Autodesk Fusion 360 part; units mm, degrees
(part 6 of 11)
  spline S6 degree 5 poles (6.7301, -111.4554) (6.7368, -111.4652) (6.7506, -111.4847) (6.7724, -111.5129) (6.8034, -111.549) (6.8449, -111.592) (6.8883, -111.6333) (6.9329, -111.6738) (6.9782, -111.7138) (7.0239, -111.7534) (7.0701, -111.7926) (7.117, -111.8312) (7.1647, -111.8691) (7.2134, -111.9062) (7.263, -111.9424) (7.3134, -111.9779) (7.3646, -112.0127) (7.4164, -112.0469) (7.4687, -112.0806) (7.5214, -112.1138) (7.5747, -112.1465) (7.6286, -112.1787) (7.6829, -112.2103) (7.7379, -112.2413) (7.7934, -112.2717) (7.8494, -112.3016) (7.9059, -112.331) (7.9629, -112.3598) (8.0204, -112.3881) (8.0782, -112.4159) (8.1365, -112.4432) (8.1952, -112.47) (8.2544, -112.4963) (8.314, -112.5221) (8.374, -112.5473) (8.4344, -112.5721) (8.4952, -112.5964) (8.5564, -112.6201) (8.6179, -112.6434) (8.6798, -112.6662) (8.7421, -112.6885) (8.8047, -112.7103) (8.8677, -112.7316) (8.9311, -112.7524) (8.9947, -112.7727) (9.0587, -112.7926) (9.1231, -112.812) (9.1877, -112.8308) (9.2527, -112.8492) (9.318, -112.8672) (9.3836, -112.8846) (9.4494, -112.9015) (9.5156, -112.918) (9.5821, -112.934) (9.6488, -112.9495) (9.7158, -112.9646) (9.7831, -112.9791) (9.8507, -112.9932) (9.9186, -113.0068) (9.9866, -113.02) (10.055, -113.0326) (10.1236, -113.0448) (10.1925, -113.0565) (10.2615, -113.0678) (10.3309, -113.0785) (10.4004, -113.0888) (10.4702, -113.0986) (10.5403, -113.108) (10.6105, -113.1168) (10.6809, -113.1252) (10.7516, -113.1331) (10.8083, -113.1391) (10.851, -113.1434) (10.8794, -113.1461) (10.8937, -113.1475) knots 0 0 0 0 0 0 0.01428571 0.02857143 0.04285714 0.05714286 0.07142857 0.08571429 0.1 0.11428571 0.12857143 0.14285714 0.15714286 0.17142857 0.18571429 0.2 0.21428571 0.22857143 0.24285714 0.25714286 0.27142857 0.28571429 0.3 0.31428571 0.32857143 0.34285714 0.35714286 0.37142857 0.38571429 0.4 0.41428571 0.42857143 0.44285714 0.45714286 0.47142857 0.48571429 0.5 0.51428571 0.52857143 0.54285714 0.55714286 0.57142857 0.58571429 0.6 0.61428571 0.62857143 0.64285714 0.65714286 0.67142857 0.68571429 0.7 0.71428571 0.72857143 0.74285714 0.75714286 0.77142857 0.78571429 0.8 0.81428571 0.82857143 0.84285714 0.85714286 0.87142857 0.88571429 0.9 0.91428571 0.92857143 0.94285714 0.95714286 0.97142857 0.98571429 1 1 1 1 1 1
  arc A14 (10.8937, -113.1475) -> (11.5475, -112.4937) centre (0, -101.6) ccw
  spline S7 degree 5 poles (11.5475, -112.4937) (11.5461, -112.4794) (11.5434, -112.451) (11.5391, -112.4083) (11.5331, -112.3516) (11.5252, -112.2809) (11.5168, -112.2105) (11.508, -112.1403) (11.4986, -112.0702) (11.4888, -112.0004) (11.4785, -111.9309) (11.4678, -111.8615) (11.4565, -111.7925) (11.4448, -111.7236) (11.4326, -111.655) (11.42, -111.5866) (11.4068, -111.5186) (11.3932, -111.4507) (11.3791, -111.3831) (11.3646, -111.3158) (11.3495, -111.2488) (11.334, -111.1821) (11.318, -111.1156) (11.3015, -111.0494) (11.2846, -110.9836) (11.2672, -110.918) (11.2492, -110.8527) (11.2308, -110.7877) (11.212, -110.7231) (11.1926, -110.6587) (11.1727, -110.5947) (11.1524, -110.5311) (11.1316, -110.4677) (11.1103, -110.4047) (11.0885, -110.3421) (11.0662, -110.2798) (11.0434, -110.2179) (11.0201, -110.1564) (10.9964, -110.0952) (10.9721, -110.0344) (10.9473, -109.974) (10.9221, -109.914) (10.8963, -109.8544) (10.87, -109.7952) (10.8432, -109.7365) (10.8159, -109.6782) (10.7881, -109.6204) (10.7598, -109.5629) (10.731, -109.5059) (10.7016, -109.4494) (10.6717, -109.3934) (10.6413, -109.3379) (10.6103, -109.2829) (10.5787, -109.2286) (10.5465, -109.1747) (10.5138, -109.1214) (10.4806, -109.0687) (10.4469, -109.0164) (10.4127, -108.9646) (10.3779, -108.9134) (10.3424, -108.863) (10.3062, -108.8134) (10.2691, -108.7647) (10.2312, -108.717) (10.1926, -108.6701) (10.1534, -108.6239) (10.1138, -108.5782) (10.0738, -108.5329) (10.0333, -108.4883) (9.992, -108.4449) (9.949, -108.4034) (9.9129, -108.3724) (9.8847, -108.3506) (9.8652, -108.3368) (9.8554, -108.3301) knots -1 -1 -1 -1 -1 -1 -0.98571429 -0.97142857 -0.95714286 -0.94285714 -0.92857143 -0.91428571 -0.9 -0.88571429 -0.87142857 -0.85714286 -0.84285714 -0.82857143 -0.81428571 -0.8 -0.78571429 -0.77142857 -0.75714286 -0.74285714 -0.72857143 -0.71428571 -0.7 -0.68571429 -0.67142857 -0.65714286 -0.64285714 -0.62857143 -0.61428571 -0.6 -0.58571429 -0.57142857 -0.55714286 -0.54285714 -0.52857143 -0.51428571 -0.5 -0.48571429 -0.47142857 -0.45714286 -0.44285714 -0.42857143 -0.41428571 -0.4 -0.38571429 -0.37142857 -0.35714286 -0.34285714 -0.32857143 -0.31428571 -0.3 -0.28571429 -0.27142857 -0.25714286 -0.24285714 -0.22857143 -0.21428571 -0.2 -0.18571429 -0.17142857 -0.15714286 -0.14285714 -0.12857143 -0.11428571 -0.1 -0.08571429 -0.07142857 -0.05714286 -0.04285714 -0.02857143 -0.01428571 0 0 0 0 0 0
  line L7 (9.8554, -108.3301) -> (8.5098, -107.41)
  arc A15 (7.9738, -105.4145) -> (8.5098, -107.41) centre (9.4058, -106.0996) ccw
  arc A16 (7.9738, -105.4145) -> (8.3356, -104.541) centre (0, -101.6) ccw
  arc A17 (10.1257, -103.509) -> (8.3356, -104.541) centre (9.8326, -105.0693) ccw
  line L8 (10.1257, -103.509) -> (11.7277, -103.8099)
  spline S8 degree 5 poles (11.7277, -103.8099) (11.7394, -103.8121) (11.7629, -103.8161) (11.7983, -103.8207) (11.8457, -103.8243) (11.9054, -103.8253) (11.9654, -103.8239) (12.0256, -103.821) (12.0858, -103.8172) (12.1462, -103.8129) (12.2066, -103.8079) (12.267, -103.8021) (12.3276, -103.7952) (12.3882, -103.7869) (12.4489, -103.7775) (12.5096, -103.7669) (12.5704, -103.7553) (12.6312, -103.7429) (12.692, -103.7298) (12.7529, -103.7159) (12.8137, -103.7014) (12.8745, -103.6861) (12.9353, -103.6699) (12.9961, -103.653) (13.0568, -103.6353) (13.1176, -103.6168) (13.1783, -103.5976) (13.2389, -103.5777) (13.2996, -103.5571) (13.3602, -103.5358) (13.4207, -103.5139) (13.4812, -103.4914) (13.5416, -103.4681) (13.602, -103.4442) (13.6622, -103.4196) (13.7225, -103.3944) (13.7826, -103.3686) (13.8427, -103.3422) (13.9026, -103.3151) (13.9625, -103.2874) (14.0223, -103.2591) (14.082, -103.2303) (14.1417, -103.2008) (14.2012, -103.1707) (14.2606, -103.1401) (14.3199, -103.1089) (14.379, -103.0771) (14.4381, -103.0447) (14.4971, -103.0118) (14.5559, -102.9783) (14.6146, -102.9442) (14.6732, -102.9096) (14.7316, -102.8745) (14.7899, -102.8388) (14.8481, -102.8026) (14.9061, -102.7658) (14.964, -102.7285) (15.0217, -102.6907) (15.0793, -102.6524) (15.1368, -102.6135) (15.194, -102.5741) (15.2512, -102.5342) (15.3081, -102.4938) (15.3649, -102.4529) (15.4216, -102.4115) (15.478, -102.3696) (15.5343, -102.3272) (15.5904, -102.2843) (15.6464, -102.2409) (15.7021, -102.197) (15.7577, -102.1526) (15.802, -102.1167) (15.8352, -102.0896) (15.8572, -102.0714) (15.8683, -102.0623) knots 0 0 0 0 0 0 0.01428571 0.02857143 0.04285714 0.05714286 0.07142857 0.08571429 0.1 0.11428571 0.12857143 0.14285714 0.15714286 0.17142857 0.18571429 0.2 0.21428571 0.22857143 0.24285714 0.25714286 0.27142857 0.28571429 0.3 0.31428571 0.32857143 0.34285714 0.35714286 0.37142857 0.38571429 0.4 0.41428571 0.42857143 0.44285714 0.45714286 0.47142857 0.48571429 0.5 0.51428571 0.52857143 0.54285714 0.55714286 0.57142857 0.58571429 0.6 0.61428571 0.62857143 0.64285714 0.65714286 0.67142857 0.68571429 0.7 0.71428571 0.72857143 0.74285714 0.75714286 0.77142857 0.78571429 0.8 0.81428571 0.82857143 0.84285714 0.85714286 0.87142857 0.88571429 0.9 0.91428571 0.92857143 0.94285714 0.95714286 0.97142857 0.98571429 1 1 1 1 1 1
  arc A18 (15.8683, -102.0623) -> (15.8683, -101.1377) centre (0, -101.6) ccw
  spline S9 degree 5 poles (15.8683, -101.1377) (15.8572, -101.1286) (15.8352, -101.1104) (15.802, -101.0833) (15.7577, -101.0474) (15.7021, -101.003) (15.6464, -100.9591) (15.5904, -100.9157) (15.5343, -100.8728) (15.478, -100.8304) (15.4216, -100.7885) (15.3649, -100.7471) (15.3081, -100.7062) (15.2512, -100.6658) (15.194, -100.6259) (15.1368, -100.5865) (15.0793, -100.5476) (15.0217, -100.5093) (14.964, -100.4715) (14.9061, -100.4342) (14.8481, -100.3974) (14.7899, -100.3612) (14.7316, -100.3255) (14.6732, -100.2904) (14.6146, -100.2558) (14.5559, -100.2217) (14.4971, -100.1882) (14.4381, -100.1553) (14.379, -100.1229) (14.3199, -100.0911) (14.2606, -100.0599) (14.2012, -100.0293) (14.1417, -99.9992) (14.082, -99.9697) (14.0223, -99.9409) (13.9625, -99.9126) (13.9026, -99.8849) (13.8427, -99.8578) (13.7826, -99.8314) (13.7225, -99.8056) (13.6622, -99.7804) (13.602, -99.7558) (13.5416, -99.7319) (13.4812, -99.7086) (13.4207, -99.6861) (13.3602, -99.6642) (13.2996, -99.6429) (13.2389, -99.6223) (13.1783, -99.6024) (13.1176, -99.5832) (13.0568, -99.5647) (12.9961, -99.547) (12.9353, -99.5301) (12.8745, -99.5139) (12.8137, -99.4986) (12.7529, -99.4841) (12.692, -99.4702) (12.6312, -99.4571) (12.5704, -99.4447) (12.5096, -99.4331) (12.4489, -99.4225) (12.3882, -99.4131) (12.3276, -99.4048) (12.267, -99.3979) (12.2066, -99.3921) (12.1462, -99.3871) (12.0858, -99.3828) (12.0256, -99.379) (11.9654, -99.3761) (11.9054, -99.3747) (11.8457, -99.3757) (11.7983, -99.3793) (11.7629, -99.3839) (11.7394, -99.3879) (11.7277, -99.3901) knots -1 -1 -1 -1 -1 -1 -0.98571429 -0.97142857 -0.95714286 -0.94285714 -0.92857143 -0.91428571 -0.9 -0.88571429 -0.87142857 -0.85714286 -0.84285714 -0.82857143 -0.81428571 -0.8 -0.78571429 -0.77142857 -0.75714286 -0.74285714 -0.72857143 -0.71428571 -0.7 -0.68571429 -0.67142857 -0.65714286 -0.64285714 -0.62857143 -0.61428571 -0.6 -0.58571429 -0.57142857 -0.55714286 -0.54285714 -0.52857143 -0.51428571 -0.5 -0.48571429 -0.47142857 -0.45714286 -0.44285714 -0.42857143 -0.41428571 -0.4 -0.38571429 -0.37142857 -0.35714286 -0.34285714 -0.32857143 -0.31428571 -0.3 -0.28571429 -0.27142857 -0.25714286 -0.24285714 -0.22857143 -0.21428571 -0.2 -0.18571429 -0.17142857 -0.15714286 -0.14285714 -0.12857143 -0.11428571 -0.1 -0.08571429 -0.07142857 -0.05714286 -0.04285714 -0.02857143 -0.01428571 0 0 0 0 0 0
  line L9 (11.7277, -99.3901) -> (10.1257, -99.691)
  arc A19 (8.3356, -98.659) -> (10.1257, -99.691) centre (9.8326, -98.1307) ccw
  arc A20 (8.3356, -98.659) -> (7.9738, -97.7855) centre (0, -101.6) ccw
  arc A21 (8.5098, -95.79) -> (7.9738, -97.7855) centre (9.4058, -97.1004) ccw
  line L10 (8.5098, -95.79) -> (9.8554, -94.8699)
  spline S10 degree 5 poles (9.8554, -94.8699) (9.8652, -94.8632) (9.8847, -94.8494) (9.9129, -94.8276) (9.949, -94.7966) (9.992, -94.7551) (10.0333, -94.7117) (10.0738, -94.6671) (10.1138, -94.6218) (10.1534, -94.5761) (10.1926, -94.5299) (10.2312, -94.483) (10.2691, -94.4353) (10.3062, -94.3866) (10.3424, -94.337) (10.3779, -94.2866) (10.4127, -94.2354) (10.4469, -94.1836) (10.4806, -94.1313) (10.5138, -94.0786) (10.5465, -94.0253) (10.5787, -93.9714) (10.6103, -93.9171) (10.6413, -93.8621) (10.6717, -93.8066) (10.7016, -93.7506) (10.731, -93.6941) (10.7598, -93.6371) (10.7881, -93.5796) (10.8159, -93.5218) (10.8432, -93.4635) (10.87, -93.4048) (10.8963, -93.3456) (10.9221, -93.286) (10.9473, -93.226) (10.9721, -93.1656) (10.9964, -93.1048) (11.0201, -93.0436) (11.0434, -92.9821) (11.0662, -92.9202) (11.0885, -92.8579) (11.1103, -92.7953) (11.1316, -92.7323) (11.1524, -92.6689) (11.1727, -92.6053) (11.1926, -92.5413) (11.212, -92.4769) (11.2308, -92.4123) (11.2492, -92.3473) (11.2672, -92.282) (11.2846, -92.2164) (11.3015, -92.1506) (11.318, -92.0844) (11.334, -92.0179) (11.3495, -91.9512) (11.3646, -91.8842) (11.3791, -91.8169) (11.3932, -91.7493) (11.4068, -91.6814) (11.42, -91.6134) (11.4326, -91.545) (11.4448, -91.4764) (11.4565, -91.4075) (11.4678, -91.3385) (11.4785, -91.2691) (11.4888, -91.1996) (11.4986, -91.1298) (11.508, -91.0597) (11.5168, -90.9895) (11.5252, -90.9191) (11.5331, -90.8484) (11.5391, -90.7917) (11.5434, -90.749) (11.5461, -90.7206) (11.5475, -90.7063) knots 0 0 0 0 0 0 0.01428571 0.02857143 0.04285714 0.05714286 0.07142857 0.08571429 0.1 0.11428571 0.12857143 0.14285714 0.15714286 0.17142857 0.18571429 0.2 0.21428571 0.22857143 0.24285714 0.25714286 0.27142857 0.28571429 0.3 0.31428571 0.32857143 0.34285714 0.35714286 0.37142857 0.38571429 0.4 0.41428571 0.42857143 0.44285714 0.45714286 0.47142857 0.48571429 0.5 0.51428571 0.52857143 0.54285714 0.55714286 0.57142857 0.58571429 0.6 0.61428571 0.62857143 0.64285714 0.65714286 0.67142857 0.68571429 0.7 0.71428571 0.72857143 0.74285714 0.75714286 0.77142857 0.78571429 0.8 0.81428571 0.82857143 0.84285714 0.85714286 0.87142857 0.88571429 0.9 0.91428571 0.92857143 0.94285714 0.95714286 0.97142857 0.98571429 1 1 1 1 1 1
  arc A22 (11.5475, -90.7063) -> (10.8937, -90.0525) centre (0, -101.6) ccw
  spline S11 degree 5 poles (10.8937, -90.0525) (10.8794, -90.0539) (10.851, -90.0566) (10.8083, -90.0609) (10.7516, -90.0669) (10.6809, -90.0748) (10.6105, -90.0832) (10.5403, -90.092) (10.4702, -90.1014) (10.4004, -90.1112) (10.3309, -90.1215) (10.2615, -90.1322) (10.1925, -90.1435) (10.1236, -90.1552) (10.055, -90.1674) (9.9866, -90.18) (9.9186, -90.1932) (9.8507, -90.2068) (9.7831, -90.2209) (9.7158, -90.2354) (9.6488, -90.2505) (9.5821, -90.266) (9.5156, -90.282) (9.4494, -90.2985) (9.3836, -90.3154) (9.318, -90.3328) (9.2527, -90.3508) (9.1877, -90.3692) (9.1231, -90.388) (9.0587, -90.4074) (8.9947, -90.4273) (8.9311, -90.4476) (8.8677, -90.4684) (8.8047, -90.4897) (8.7421, -90.5115) (8.6798, -90.5338) (8.6179, -90.5566) (8.5564, -90.5799) (8.4952, -90.6036) (8.4344, -90.6279) (8.374, -90.6527) (8.314, -90.6779) (8.2544, -90.7037) (8.1952, -90.73) (8.1365, -90.7568) (8.0782, -90.7841) (8.0204, -90.8119) (7.9629, -90.8402) (7.9059, -90.869) (7.8494, -90.8984) (7.7934, -90.9283) (7.7379, -90.9587) (7.6829, -90.9897) (7.6286, -91.0213) (7.5747, -91.0535) (7.5214, -91.0862) (7.4687, -91.1194) (7.4164, -91.1531) (7.3646, -91.1873) (7.3134, -91.2221) (7.263, -91.2576) (7.2134, -91.2938) (7.1647, -91.3309) (7.117, -91.3688) (7.0701, -91.4074) (7.0239, -91.4466) (6.9782, -91.4862) (6.9329, -91.5262) (6.8883, -91.5667) (6.8449, -91.608) (6.8034, -91.651) (6.7724, -91.6871) (6.7506, -91.7153) (6.7368, -91.7348) (6.7301, -91.7446) knots -1 -1 -1 -1 -1 -1 -0.98571429 -0.97142857 -0.95714286 -0.94285714 -0.92857143 -0.91428571 -0.9 -0.88571429 -0.87142857 -0.85714286 -0.84285714 -0.82857143 -0.81428571 -0.8 -0.78571429 -0.77142857 -0.75714286 -0.74285714 -0.72857143 -0.71428571 -0.7 -0.68571429 -0.67142857 -0.65714286 -0.64285714 -0.62857143 -0.61428571 -0.6 -0.58571429 -0.57142857 -0.55714286 -0.54285714 -0.52857143 -0.51428571 -0.5 -0.48571429 -0.47142857 -0.45714286 -0.44285714 -0.42857143 -0.41428571 -0.4 -0.38571429 -0.37142857 -0.35714286 -0.34285714 -0.32857143 -0.31428571 -0.3 -0.28571429 -0.27142857 -0.25714286 -0.24285714 -0.22857143 -0.21428571 -0.2 -0.18571429 -0.17142857 -0.15714286 -0.14285714 -0.12857143 -0.11428571 -0.1 -0.08571429 -0.07142857 -0.05714286 -0.04285714 -0.02857143 -0.01428571 0 0 0 0 0 0
  line L11 (6.7301, -91.7446) -> (5.81, -93.0902)
  arc A23 (3.8145, -93.6262) -> (5.81, -93.0902) centre (4.4996, -92.1942) ccw
  arc A24 (3.8145, -93.6262) -> (2.941, -93.2644) centre (0, -101.6) ccw
  arc A25 (1.909, -91.4743) -> (2.941, -93.2644) centre (3.4693, -91.7674) ccw
  line L12 (1.909, -91.4743) -> (2.2099, -89.8723)
  spline S12 degree 5 poles (2.2099, -89.8723) (2.2121, -89.8606) (2.2161, -89.8371) (2.2207, -89.8017) (2.2243, -89.7543) (2.2253, -89.6946) (2.2239, -89.6346) (2.221, -89.5744) (2.2172, -89.5142) (2.2129, -89.4538) (2.2079, -89.3934) (2.2021, -89.333) (2.1952, -89.2724) (2.1869, -89.2118) (2.1775, -89.1511) (2.1669, -89.0904) (2.1553, -89.0296) (2.1429, -88.9688) (2.1298, -88.908) (2.1159, -88.8471) (2.1014, -88.7863) (2.0861, -88.7255) (2.0699, -88.6647) (2.053, -88.6039) (2.0353, -88.5432) (2.0168, -88.4824) (1.9976, -88.4217) (1.9777, -88.3611) (1.9571, -88.3004) (1.9358, -88.2398) (1.9139, -88.1793) (1.8914, -88.1188) (1.8681, -88.0584) (1.8442, -87.998) (1.8196, -87.9378) (1.7944, -87.8775) (1.7686, -87.8174) (1.7422, -87.7573) (1.7151, -87.6974) (1.6874, -87.6375) (1.6591, -87.5777) (1.6303, -87.518) (1.6008, -87.4583) (1.5707, -87.3988) (1.5401, -87.3394) (1.5089, -87.2801) (1.4771, -87.221) (1.4447, -87.1619) (1.4118, -87.1029) (1.3783, -87.0441) (1.3442, -86.9854) (1.3096, -86.9268) (1.2745, -86.8684) (1.2388, -86.8101) (1.2026, -86.7519) (1.1658, -86.6939) (1.1285, -86.636) (1.0907, -86.5783) (1.0524, -86.5207) (1.0135, -86.4632) (0.9741, -86.406) (0.9342, -86.3488) (0.8938, -86.2919) (0.8529, -86.2351) (0.8115, -86.1784) (0.7696, -86.122) (0.7272, -86.0657) (0.6843, -86.0096) (0.6409, -85.9536) (0.597, -85.8979) (0.5526, -85.8423) (0.5167, -85.798) (0.4896, -85.7648) (0.4714, -85.7428) (0.4623, -85.7317) knots 0 0 0 0 0 0 0.01428571 0.02857143 0.04285714 0.05714286 0.07142857 0.08571429 0.1 0.11428571 0.12857143 0.14285714 0.15714286 0.17142857 0.18571429 0.2 0.21428571 0.22857143 0.24285714 0.25714286 0.27142857 0.28571429 0.3 0.31428571 0.32857143 0.34285714 0.35714286 0.37142857 0.38571429 0.4 0.41428571 0.42857143 0.44285714 0.45714286 0.47142857 0.48571429 0.5 0.51428571 0.52857143 0.54285714 0.55714286 0.57142857 0.58571429 0.6 0.61428571 0.62857143 0.64285714 0.65714286 0.67142857 0.68571429 0.7 0.71428571 0.72857143 0.74285714 0.75714286 0.77142857 0.78571429 0.8 0.81428571 0.82857143 0.84285714 0.85714286 0.87142857 0.88571429 0.9 0.91428571 0.92857143 0.94285714 0.95714286 0.97142857 0.98571429 1 1 1 1 1 1
  arc A26 (0.4623, -85.7317) -> (-0.4623, -85.7317) centre (0, -101.6) ccw
  spline S13 degree 5 poles (-0.4623, -85.7317) (-0.4714, -85.7428) (-0.4896, -85.7648) (-0.5167, -85.798) (-0.5526, -85.8423) (-0.597, -85.8979) (-0.6409, -85.9536) (-0.6843, -86.0096) (-0.7272, -86.0657) (-0.7696, -86.122) (-0.8115, -86.1784) (-0.8529, -86.2351) (-0.8938, -86.2919) (-0.9342, -86.3488) (-0.9741, -86.406) (-1.0135, -86.4632) (-1.0524, -86.5207) (-1.0907, -86.5783) (-1.1285, -86.636) (-1.1658, -86.6939) (-1.2026, -86.7519) (-1.2388, -86.8101) (-1.2745, -86.8684) (-1.3096, -86.9268) (-1.3442, -86.9854) (-1.3783, -87.0441) (-1.4118, -87.1029) (-1.4447, -87.1619) (-1.4771, -87.221) (-1.5089, -87.2801) (-1.5401, -87.3394) (-1.5707, -87.3988) (-1.6008, -87.4583) (-1.6303, -87.518) (-1.6591, -87.5777) (-1.6874, -87.6375) (-1.7151, -87.6974) (-1.7422, -87.7573) (-1.7686, -87.8174) (-1.7944, -87.8775) (-1.8196, -87.9378) (-1.8442, -87.998) (-1.8681, -88.0584) (-1.8914, -88.1188) (-1.9139, -88.1793) (-1.9358, -88.2398) (-1.9571, -88.3004) (-1.9777, -88.3611) (-1.9976, -88.4217) (-2.0168, -88.4824) (-2.0353, -88.5432) (-2.053, -88.6039) (-2.0699, -88.6647) (-2.0861, -88.7255) (-2.1014, -88.7863) (-2.1159, -88.8471) (-2.1298, -88.908) (-2.1429, -88.9688) (-2.1553, -89.0296) (-2.1669, -89.0904) (-2.1775, -89.1511) (-2.1869, -89.2118) (-2.1952, -89.2724) (-2.2021, -89.333) (-2.2079, -89.3934) (-2.2129, -89.4538) (-2.2172, -89.5142) (-2.221, -89.5744) (-2.2239, -89.6346) (-2.2253, -89.6946) (-2.2243, -89.7543) (-2.2207, -89.8017) (-2.2161, -89.8371) (-2.2121, -89.8606) (-2.2099, -89.8723) knots -1 -1 -1 -1 -1 -1 -0.98571429 -0.97142857 -0.95714286 -0.94285714 -0.92857143 -0.91428571 -0.9 -0.88571429 -0.87142857 -0.85714286 -0.84285714 -0.82857143 -0.81428571 -0.8 -0.78571429 -0.77142857 -0.75714286 -0.74285714 -0.72857143 -0.71428571 -0.7 -0.68571429 -0.67142857 -0.65714286 -0.64285714 -0.62857143 -0.61428571 -0.6 -0.58571429 -0.57142857 -0.55714286 -0.54285714 -0.52857143 -0.51428571 -0.5 -0.48571429 -0.47142857 -0.45714286 -0.44285714 -0.42857143 -0.41428571 -0.4 -0.38571429 -0.37142857 -0.35714286 -0.34285714 -0.32857143 -0.31428571 -0.3 -0.28571429 -0.27142857 -0.25714286 -0.24285714 -0.22857143 -0.21428571 -0.2 -0.18571429 -0.17142857 -0.15714286 -0.14285714 -0.12857143 -0.11428571 -0.1 -0.08571429 -0.07142857 -0.05714286 -0.04285714 -0.02857143 -0.01428571 0 0 0 0 0 0
  line L13 (-2.2099, -89.8723) -> (-1.909, -91.4743)
  arc A27 (-2.941, -93.2644) -> (-1.909, -91.4743) centre (-3.4693, -91.7674) ccw
  arc A28 (-2.941, -93.2644) -> (-3.8145, -93.6262) centre (0, -101.6) ccw
  arc A29 (-5.81, -93.0902) -> (-3.8145, -93.6262) centre (-4.4996, -92.1942) ccw
  line L14 (-5.81, -93.0902) -> (-6.7301, -91.7446)
  spline S14 degree 5 poles (-6.7301, -91.7446) (-6.7368, -91.7348) (-6.7506, -91.7153) (-6.7724, -91.6871) (-6.8034, -91.651) (-6.8449, -91.608) (-6.8883, -91.5667) (-6.9329, -91.5262) (-6.9782, -91.4862) (-7.0239, -91.4466) (-7.0701, -91.4074) (-7.117, -91.3688) (-7.1647, -91.3309) (-7.2134, -91.2938) (-7.263, -91.2576) (-7.3134, -91.2221) (-7.3646, -91.1873) (-7.4164, -91.1531) (-7.4687, -91.1194) (-7.5214, -91.0862) (-7.5747, -91.0535) (-7.6286, -91.0213) (-7.6829, -90.9897) (-7.7379, -90.9587) (-7.7934, -90.9283) (-7.8494, -90.8984) (-7.9059, -90.869) (-7.9629, -90.8402) (-8.0204, -90.8119) (-8.0782, -90.7841) (-8.1365, -90.7568) (-8.1952, -90.73) (-8.2544, -90.7037) (-8.314, -90.6779) (-8.374, -90.6527) (-8.4344, -90.6279) (-8.4952, -90.6036) (-8.5564, -90.5799) (-8.6179, -90.5566) (-8.6798, -90.5338) (-8.7421, -90.5115) (-8.8047, -90.4897) (-8.8677, -90.4684) (-8.9311, -90.4476) (-8.9947, -90.4273) (-9.0587, -90.4074) (-9.1231, -90.388) (-9.1877, -90.3692) (-9.2527, -90.3508) (-9.318, -90.3328) (-9.3836, -90.3154) (-9.4494, -90.2985) (-9.5156, -90.282) (-9.5821, -90.266) (-9.6488, -90.2505) (-9.7158, -90.2354) (-9.7831, -90.2209) (-9.8507, -90.2068) (-9.9186, -90.1932) (-9.9866, -90.18) (-10.055, -90.1674) (-10.1236, -90.1552) (-10.1925, -90.1435) (-10.2615, -90.1322) (-10.3309, -90.1215) (-10.4004, -90.1112) (-10.4702, -90.1014) (-10.5403, -90.092) (-10.6105, -90.0832) (-10.6809, -90.0748) (-10.7516, -90.0669) (-10.8083, -90.0609) (-10.851, -90.0566) (-10.8794, -90.0539) (-10.8937, -90.0525) knots 0 0 0 0 0 0 0.01428571 0.02857143 0.04285714 0.05714286 0.07142857 0.08571429 0.1 0.11428571 0.12857143 0.14285714 0.15714286 0.17142857 0.18571429 0.2 0.21428571 0.22857143 0.24285714 0.25714286 0.27142857 0.28571429 0.3 0.31428571 0.32857143 0.34285714 0.35714286 0.37142857 0.38571429 0.4 0.41428571 0.42857143 0.44285714 0.45714286 0.47142857 0.48571429 0.5 0.51428571 0.52857143 0.54285714 0.55714286 0.57142857 0.58571429 0.6 0.61428571 0.62857143 0.64285714 0.65714286 0.67142857 0.68571429 0.7 0.71428571 0.72857143 0.74285714 0.75714286 0.77142857 0.78571429 0.8 0.81428571 0.82857143 0.84285714 0.85714286 0.87142857 0.88571429 0.9 0.91428571 0.92857143 0.94285714 0.95714286 0.97142857 0.98571429 1 1 1 1 1 1
  arc A30 (-10.8937, -90.0525) -> (-11.5475, -90.7063) centre (0, -101.6) ccw
  spline S15 degree 5 poles (-11.5475, -90.7063) (-11.5461, -90.7206) (-11.5434, -90.749) (-11.5391, -90.7917) (-11.5331, -90.8484) (-11.5252, -90.9191) (-11.5168, -90.9895) (-11.508, -91.0597) (-11.4986, -91.1298) (-11.4888, -91.1996) (-11.4785, -91.2691) (-11.4678, -91.3385) (-11.4565, -91.4075) (-11.4448, -91.4764) (-11.4326, -91.545) (-11.42, -91.6134) (-11.4068, -91.6814) (-11.3932, -91.7493) (-11.3791, -91.8169) (-11.3646, -91.8842) (-11.3495, -91.9512) (-11.334, -92.0179) (-11.318, -92.0844) (-11.3015, -92.1506) (-11.2846, -92.2164) (-11.2672, -92.282) (-11.2492, -92.3473) (-11.2308, -92.4123) (-11.212, -92.4769) (-11.1926, -92.5413) (-11.1727, -92.6053) (-11.1524, -92.6689) (-11.1316, -92.7323) (-11.1103, -92.7953) (-11.0885, -92.8579) (-11.0662, -92.9202) (-11.0434, -92.9821) (-11.0201, -93.0436) (-10.9964, -93.1048) (-10.9721, -93.1656) (-10.9473, -93.226) (-10.9221, -93.286) (-10.8963, -93.3456) (-10.87, -93.4048) (-10.8432, -93.4635) (-10.8159, -93.5218) (-10.7881, -93.5796) (-10.7598, -93.6371) (-10.731, -93.6941) (-10.7016, -93.7506) (-10.6717, -93.8066) (-10.6413, -93.8621) (-10.6103, -93.9171) (-10.5787, -93.9714) (-10.5465, -94.0253) (-10.5138, -94.0786) (-10.4806, -94.1313) (-10.4469, -94.1836) (-10.4127, -94.2354) (-10.3779, -94.2866) (-10.3424, -94.337) (-10.3062, -94.3866) (-10.2691, -94.4353) (-10.2312, -94.483) (-10.1926, -94.5299) (-10.1534, -94.5761) (-10.1138, -94.6218) (-10.0738, -94.6671) (-10.0333, -94.7117) (-9.992, -94.7551) (-9.949, -94.7966) (-9.9129, -94.8276) (-9.8847, -94.8494) (-9.8652, -94.8632) (-9.8554, -94.8699) knots -1 -1 -1 -1 -1 -1 -0.98571429 -0.97142857 -0.95714286 -0.94285714 -0.92857143 -0.91428571 -0.9 -0.88571429 -0.87142857 -0.85714286 -0.84285714 -0.82857143 -0.81428571 -0.8 -0.78571429 -0.77142857 -0.75714286 -0.74285714 -0.72857143 -0.71428571 -0.7 -0.68571429 -0.67142857 -0.65714286 -0.64285714 -0.62857143 -0.61428571 -0.6 -0.58571429 -0.57142857 -0.55714286 -0.54285714 -0.52857143 -0.51428571 -0.5 -0.48571429 -0.47142857 -0.45714286 -0.44285714 -0.42857143 -0.41428571 -0.4 -0.38571429 -0.37142857 -0.35714286 -0.34285714 -0.32857143 -0.31428571 -0.3 -0.28571429 -0.27142857 -0.25714286 -0.24285714 -0.22857143 -0.21428571 -0.2 -0.18571429 -0.17142857 -0.15714286 -0.14285714 -0.12857143 -0.11428571 -0.1 -0.08571429 -0.07142857 -0.05714286 -0.04285714 -0.02857143 -0.01428571 0 0 0 0 0 0
  line L15 (-9.8554, -94.8699) -> (-8.5098, -95.79)
  arc A31 (-7.9738, -97.7855) -> (-8.5098, -95.79) centre (-9.4058, -97.1004) ccw
  circle A32 centre (0, -101.6) radius 6.35
  circle A33 centre (0, -101.6) radius 6.35
  constraint concentric A0 A33
extrude "Extrude1''" add sketch "Sketch2 (3)" along normal mid plane 35.56 separate body contours A96 A97 makes body 3
extrude "Extrude2''" add sketch "Sketch3 (3)" along normal mid plane 35.56 separate body contours A64 A65 makes body 4
extrude "Extrude3" add sketch "Sketch4" along normal mid plane 35.56 separate body contours A32 A33 makes body 5
copy_body "Body->Comp1" bodies 3 removing the originals makes body 6 in component "Component"
copy_body "Body->Comp2" bodies 4 removing the originals makes body 7 in component "Component'"
copy_body "Body->Comp3" bodies 5 removing the originals makes body 8 in component "Component''"
sketch "Sketch1 (3)" plane through (0, 0, 0) normal (0, 0, 1) x (1, 0, 0) in component "Spur Gear (8 teeth)"
  circle A0 centre (0, 0) radius 8.8392
  circle A1 centre (0, 0) radius 6.35
extrude "Extrude1'''" add sketch "Sketch1 (3)" along normal blind 12.7 separate body makes body 9 in component "Spur Gear (8 teeth)"
sketch "Sketch2 (4)" plane through (0, 0, 0) normal (0, 0, 1) x (1, 0, 0) in component "Spur Gear (8 teeth)"
  spline S0 degree 5 poles (11.6688, -2.5024) (11.6805, -2.5049) (11.7038, -2.5094) (11.7391, -2.5149) (11.7864, -2.5197) (11.8461, -2.5222) (11.9061, -2.5223) (11.9663, -2.5209) (12.0266, -2.5186) (12.087, -2.5158) (12.1476, -2.5124) (12.2081, -2.5081) (12.2688, -2.5026) (12.3297, -2.4959) (12.3906, -2.488) (12.4516, -2.4789) (12.5126, -2.4689) (12.5737, -2.458) (12.6348, -2.4464) (12.696, -2.4341) (12.7571, -2.421) (12.8183, -2.4072) (12.8795, -2.3926) (12.9407, -2.3772) (13.0019, -2.361) (13.063, -2.3441) (13.1242, -2.3264) (13.1854, -2.308) (13.2465, -2.2889) (13.3076, -2.2692) (13.3687, -2.2488) (13.4297, -2.2278) (13.4907, -2.206) (13.5516, -2.1836) (13.6125, -2.1606) (13.6733, -2.1369) (13.7341, -2.1126) (13.7948, -2.0876) (13.8554, -2.0621) (13.916, -2.0359) (13.9765, -2.0091) (14.0369, -1.9818) (14.0972, -1.9538) (14.1575, -1.9252) (14.2176, -1.8961) (14.2777, -1.8663) (14.3376, -1.836) (14.3975, -1.8052) (14.4572, -1.7737) (14.5169, -1.7417) (14.5764, -1.7091) (14.6358, -1.676) (14.6951, -1.6424) (14.7543, -1.6081) (14.8134, -1.5734) (14.8723, -1.5381) (14.9311, -1.5022) (14.9898, -1.4659) (15.0483, -1.429) (15.1067, -1.3916) (15.1649, -1.3536) (15.2231, -1.3152) (15.281, -1.2762) (15.3388, -1.2367) (15.3965, -1.1968) (15.454, -1.1563) (15.5113, -1.1153) (15.5685, -1.0738) (15.6255, -1.0318) (15.6823, -0.9893) (15.739, -0.9464) (15.7842, -0.9116) (15.818, -0.8853) (15.8405, -0.8677) (15.8518, -0.8588) knots 0 0 0 0 0 0 0.01428571 0.02857143 0.04285714 0.05714286 0.07142857 0.08571429 0.1 0.11428571 0.12857143 0.14285714 0.15714286 0.17142857 0.18571429 0.2 0.21428571 0.22857143 0.24285714 0.25714286 0.27142857 0.28571429 0.3 0.31428571 0.32857143 0.34285714 0.35714286 0.37142857 0.38571429 0.4 0.41428571 0.42857143 0.44285714 0.45714286 0.47142857 0.48571429 0.5 0.51428571 0.52857143 0.54285714 0.55714286 0.57142857 0.58571429 0.6 0.61428571 0.62857143 0.64285714 0.65714286 0.67142857 0.68571429 0.7 0.71428571 0.72857143 0.74285714 0.75714286 0.77142857 0.78571429 0.8 0.81428571 0.82857143 0.84285714 0.85714286 0.87142857 0.88571429 0.9 0.91428571 0.92857143 0.94285714 0.95714286 0.97142857 0.98571429 1 1 1 1 1 1
  spline S1 degree 5 poles (11.6688, 2.5024) (11.6805, 2.5049) (11.7038, 2.5094) (11.7391, 2.5149) (11.7864, 2.5197) (11.8461, 2.5222) (11.9061, 2.5223) (11.9663, 2.5209) (12.0266, 2.5186) (12.087, 2.5158) (12.1476, 2.5124) (12.2081, 2.5081) (12.2688, 2.5026) (12.3297, 2.4959) (12.3906, 2.488) (12.4516, 2.4789) (12.5126, 2.4689) (12.5737, 2.458) (12.6348, 2.4464) (12.696, 2.4341) (12.7571, 2.421) (12.8183, 2.4072) (12.8795, 2.3926) (12.9407, 2.3772) (13.0019, 2.361) (13.063, 2.3441) (13.1242, 2.3264) (13.1854, 2.308) (13.2465, 2.2889) (13.3076, 2.2692) (13.3687, 2.2488) (13.4297, 2.2278) (13.4907, 2.206) (13.5516, 2.1836) (13.6125, 2.1606) (13.6733, 2.1369) (13.7341, 2.1126) (13.7948, 2.0876) (13.8554, 2.0621) (13.916, 2.0359) (13.9765, 2.0091) (14.0369, 1.9818) (14.0972, 1.9538) (14.1575, 1.9252) (14.2176, 1.8961) (14.2777, 1.8663) (14.3376, 1.836) (14.3975, 1.8052) (14.4572, 1.7737) (14.5169, 1.7417) (14.5764, 1.7091) (14.6358, 1.676) (14.6951, 1.6424) (14.7543, 1.6081) (14.8134, 1.5734) (14.8723, 1.5381) (14.9311, 1.5022) (14.9898, 1.4659) (15.0483, 1.429) (15.1067, 1.3916) (15.1649, 1.3536) (15.2231, 1.3152) (15.281, 1.2762) (15.3388, 1.2367) (15.3965, 1.1968) (15.454, 1.1563) (15.5113, 1.1153) (15.5685, 1.0738) (15.6255, 1.0318) (15.6823, 0.9893) (15.739, 0.9464) (15.7842, 0.9116) (15.818, 0.8853) (15.8405, 0.8677) (15.8518, 0.8588) knots 0 0 0 0 0 0 0.01428571 0.02857143 0.04285714 0.05714286 0.07142857 0.08571429 0.1 0.11428571 0.12857143 0.14285714 0.15714286 0.17142857 0.18571429 0.2 0.21428571 0.22857143 0.24285714 0.25714286 0.27142857 0.28571429 0.3 0.31428571 0.32857143 0.34285714 0.35714286 0.37142857 0.38571429 0.4 0.41428571 0.42857143 0.44285714 0.45714286 0.47142857 0.48571429 0.5 0.51428571 0.52857143 0.54285714 0.55714286 0.57142857 0.58571429 0.6 0.61428571 0.62857143 0.64285714 0.65714286 0.67142857 0.68571429 0.7 0.71428571 0.72857143 0.74285714 0.75714286 0.77142857 0.78571429 0.8 0.81428571 0.82857143 0.84285714 0.85714286 0.87142857 0.88571429 0.9 0.91428571 0.92857143 0.94285714 0.95714286 0.97142857 0.98571429 1 1 1 1 1 1
  arc A0 (15.8518, -0.8588) -> (15.8518, 0.8588) centre (0, 0) ccw
  line L0 (8.6329, -1.8535) -> (11.6688, -2.5024)
  line L1 (8.6329, 1.8535) -> (11.6688, 2.5024)
  line L2 (8.6329, -1.8535) -> (8.6329, 1.8535)
  point P0 (11.9526, -2.5211)
  point P1 (12.2435, -2.5047)
  point P2 (12.5387, -2.4641)
  point P3 (12.8372, -2.4026)
  point P4 (13.1379, -2.3222)
  point P5 (13.4403, -2.2238)
  point P6 (13.7438, -2.1085)
  point P7 (14.0477, -1.9767)
  point P8 (14.3515, -1.8288)
  point P9 (14.6547, -1.6652)
  point P10 (14.9569, -1.4862)
  point P11 (15.2574, -1.292)
  point P12 (15.5559, -1.0828)
  point P13 (11.9526, 2.5211)
  point P14 (12.2435, 2.5047)
  point P15 (12.5387, 2.4641)
  point P16 (12.8372, 2.4026)
  point P17 (13.1379, 2.3222)
  point P18 (13.4403, 2.2238)
  point P19 (13.7438, 2.1085)
  point P20 (14.0477, 1.9767)
  point P21 (14.3515, 1.8288)
  point P22 (14.6547, 1.6652)
  point P23 (14.9569, 1.4862)
  point P24 (15.2574, 1.292)
  point P25 (15.5559, 1.0828)
extrude "Extrude2'''" add sketch "Sketch2 (4)" along normal blind 12.7 bodies 9 in component "Spur Gear (8 teeth)"
fillet "Fillet1''" radius 1.0922 2 edges at (8.6423, -1.8555, 6.35) (8.6423, 1.8555, 6.35) on bodies 9 in component "Spur Gear (8 teeth)"
pattern_circular "C-Pattern1''" count 8 over 360 about axis through (0, 0, 0) along (0, 0, 1) of "Extrude2'''", "Fillet1''" in component "Spur Gear (8 teeth)"
sketch "Sketch3 (4)" plane through (0, 0, 0) normal (0, 0, 1) x (1, 0, 0) in component "Spur Gear (8 teeth)"
  circle A0 centre (0, 0) radius 12.7 construction
sketch "Sketch5" plane through (0, 0, 12.7) normal (0, 0, 1) x (-1, 0, 0)
  arc A0 (-33.9178, 4.6802) -> (-33.9734, 4.2579) centre (0, 0) ccw
  arc A1 (-35.6752, 2.8728) -> (-33.9734, 4.2579) centre (-35.5486, 4.4553) ccw
  line L0 (-35.6752, 2.8728) -> (-35.6868, 2.8738)
  spline S0 degree 5 poles (-35.6868, 2.8738) (-35.7028, 2.8751) (-35.735, 2.8772) (-35.7832, 2.8793) (-35.8475, 2.8797) (-35.9281, 2.8771) (-36.0087, 2.8722) (-36.0893, 2.8659) (-36.17, 2.8589) (-36.2507, 2.8513) (-36.3314, 2.8432) (-36.4121, 2.8344) (-36.4928, 2.8246) (-36.5735, 2.8138) (-36.6542, 2.8018) (-36.7349, 2.7889) (-36.8156, 2.775) (-36.8963, 2.7604) (-36.9769, 2.7452) (-37.0576, 2.7294) (-37.1382, 2.713) (-37.2187, 2.696) (-37.2993, 2.6783) (-37.3798, 2.6599) (-37.4603, 2.6409) (-37.5408, 2.6212) (-37.6212, 2.6008) (-37.7016, 2.5799) (-37.7819, 2.5584) (-37.8622, 2.5364) (-37.9425, 2.5139) (-38.0227, 2.4907) (-38.1029, 2.4671) (-38.183, 2.4429) (-38.2631, 2.4181) (-38.3431, 2.3929) (-38.4231, 2.3671) (-38.503, 2.3408) (-38.5829, 2.314) (-38.6627, 2.2867) (-38.7425, 2.2589) (-38.8222, 2.2307) (-38.9018, 2.2019) (-38.9814, 2.1727) (-39.061, 2.143) (-39.1404, 2.1129) (-39.2198, 2.0822) (-39.2992, 2.0512) (-39.3785, 2.0196) (-39.4577, 1.9876) (-39.5369, 1.9552) (-39.6159, 1.9224) (-39.695, 1.889) (-39.7739, 1.8553) (-39.8528, 1.8211) (-39.9316, 1.7865) (-40.0103, 1.7515) (-40.089, 1.7161) (-40.1676, 1.6802) (-40.2461, 1.644) (-40.3245, 1.6073) (-40.4029, 1.5702) (-40.4811, 1.5327) (-40.5593, 1.4948) (-40.6374, 1.4565) (-40.7155, 1.4178) (-40.7934, 1.3787) (-40.8713, 1.3392) (-40.9491, 1.2993) (-41.0268, 1.259) (-41.1044, 1.2184) (-41.1664, 1.1855) (-41.2129, 1.1607) (-41.2439, 1.1441) (-41.2594, 1.1358) knots 0 0 0 0 0 0 0.01428571 0.02857143 0.04285714 0.05714286 0.07142857 0.08571429 0.1 0.11428571 0.12857143 0.14285714 0.15714286 0.17142857 0.18571429 0.2 0.21428571 0.22857143 0.24285714 0.25714286 0.27142857 0.28571429 0.3 0.31428571 0.32857143 0.34285714 0.35714286 0.37142857 0.38571429 0.4 0.41428571 0.42857143 0.44285714 0.45714286 0.47142857 0.48571429 0.5 0.51428571 0.52857143 0.54285714 0.55714286 0.57142857 0.58571429 0.6 0.61428571 0.62857143 0.64285714 0.65714286 0.67142857 0.68571429 0.7 0.71428571 0.72857143 0.74285714 0.75714286 0.77142857 0.78571429 0.8 0.81428571 0.82857143 0.84285714 0.85714286 0.87142857 0.88571429 0.9 0.91428571 0.92857143 0.94285714 0.95714286 0.97142857 0.98571429 1 1 1 1 1 1
  arc A2 (-41.2594, 1.1358) -> (-41.2594, -1.1358) centre (0, 0) ccw
  spline S1 degree 5 poles (-41.2594, -1.1358) (-41.2439, -1.1441) (-41.2129, -1.1607) (-41.1664, -1.1855) (-41.1044, -1.2184) (-41.0268, -1.259) (-40.9491, -1.2993) (-40.8713, -1.3392) (-40.7934, -1.3787) (-40.7155, -1.4178) (-40.6374, -1.4565) (-40.5593, -1.4948) (-40.4811, -1.5327) (-40.4029, -1.5702) (-40.3245, -1.6073) (-40.2461, -1.644) (-40.1676, -1.6802) (-40.089, -1.7161) (-40.0103, -1.7515) (-39.9316, -1.7865) (-39.8528, -1.8211) (-39.7739, -1.8553) (-39.695, -1.889) (-39.6159, -1.9224) (-39.5369, -1.9552) (-39.4577, -1.9876) (-39.3785, -2.0196) (-39.2992, -2.0512) (-39.2198, -2.0822) (-39.1404, -2.1129) (-39.061, -2.143) (-38.9814, -2.1727) (-38.9018, -2.2019) (-38.8222, -2.2307) (-38.7425, -2.2589) (-38.6627, -2.2867) (-38.5829, -2.314) (-38.503, -2.3408) (-38.4231, -2.3671) (-38.3431, -2.3929) (-38.2631, -2.4181) (-38.183, -2.4429) (-38.1029, -2.4671) (-38.0227, -2.4907) (-37.9425, -2.5139) (-37.8622, -2.5364) (-37.7819, -2.5584) (-37.7016, -2.5799) (-37.6212, -2.6008) (-37.5408, -2.6212) (-37.4603, -2.6409) (-37.3798, -2.6599) (-37.2993, -2.6783) (-37.2187, -2.696) (-37.1382, -2.713) (-37.0576, -2.7294) (-36.9769, -2.7452) (-36.8963, -2.7604) (-36.8156, -2.775) (-36.7349, -2.7889) (-36.6542, -2.8018) (-36.5735, -2.8138) (-36.4928, -2.8246) (-36.4121, -2.8344) (-36.3314, -2.8432) (-36.2507, -2.8513) (-36.17, -2.8589) (-36.0893, -2.8659) (-36.0087, -2.8722) (-35.9281, -2.8771) (-35.8475, -2.8797) (-35.7832, -2.8793) (-35.735, -2.8772) (-35.7028, -2.8751) (-35.6868, -2.8738) knots -1 -1 -1 -1 -1 -1 -0.98571429 -0.97142857 -0.95714286 -0.94285714 -0.92857143 -0.91428571 -0.9 -0.88571429 -0.87142857 -0.85714286 -0.84285714 -0.82857143 -0.81428571 -0.8 -0.78571429 -0.77142857 -0.75714286 -0.74285714 -0.72857143 -0.71428571 -0.7 -0.68571429 -0.67142857 -0.65714286 -0.64285714 -0.62857143 -0.61428571 -0.6 -0.58571429 -0.57142857 -0.55714286 -0.54285714 -0.52857143 -0.51428571 -0.5 -0.48571429 -0.47142857 -0.45714286 -0.44285714 -0.42857143 -0.41428571 -0.4 -0.38571429 -0.37142857 -0.35714286 -0.34285714 -0.32857143 -0.31428571 -0.3 -0.28571429 -0.27142857 -0.25714286 -0.24285714 -0.22857143 -0.21428571 -0.2 -0.18571429 -0.17142857 -0.15714286 -0.14285714 -0.12857143 -0.11428571 -0.1 -0.08571429 -0.07142857 -0.05714286 -0.04285714 -0.02857143 -0.01428571 0 0 0 0 0 0
  line L1 (-35.6868, -2.8738) -> (-35.6752, -2.8728)
  arc A3 (-33.9734, -4.2579) -> (-35.6752, -2.8728) centre (-35.5486, -4.4553) ccw
  arc A4 (-33.9734, -4.2579) -> (-33.9178, -4.6802) centre (0, 0) ccw
  arc A5 (-35.2032, -6.4585) -> (-33.9178, -4.6802) centre (-35.4904, -4.8972) ccw
  line L2 (-35.2032, -6.4585) -> (-35.2146, -6.4606)
  spline S2 degree 5 poles (-35.2146, -6.4606) (-35.2304, -6.4635) (-35.262, -6.4697) (-35.3091, -6.4802) (-35.3714, -6.4965) (-35.4485, -6.5198) (-35.5251, -6.5454) (-35.6014, -6.5723) (-35.6775, -6.6) (-35.7535, -6.6282) (-35.8293, -6.6569) (-35.905, -6.6863) (-35.9804, -6.7167) (-36.0556, -6.748) (-36.1304, -6.7805) (-36.205, -6.8139) (-36.2794, -6.8481) (-36.3535, -6.8831) (-36.4275, -6.9186) (-36.5013, -6.9548) (-36.5749, -6.9915) (-36.6483, -7.0288) (-36.7215, -7.0667) (-36.7946, -7.1053) (-36.8674, -7.1446) (-36.94, -7.1844) (-37.0124, -7.2249) (-37.0846, -7.2659) (-37.1567, -7.3074) (-37.2286, -7.3495) (-37.3002, -7.392) (-37.3717, -7.4351) (-37.4431, -7.4787) (-37.5142, -7.5228) (-37.5851, -7.5675) (-37.6559, -7.6126) (-37.7265, -7.6582) (-37.7969, -7.7043) (-37.8671, -7.7508) (-37.9371, -7.7979) (-38.007, -7.8453) (-38.0767, -7.8933) (-38.1462, -7.9416) (-38.2155, -7.9905) (-38.2846, -8.0397) (-38.3536, -8.0894) (-38.4224, -8.1396) (-38.491, -8.1901) (-38.5594, -8.2411) (-38.6277, -8.2925) (-38.6957, -8.3443) (-38.7636, -8.3965) (-38.8313, -8.4491) (-38.8988, -8.5022) (-38.9662, -8.5556) (-39.0333, -8.6094) (-39.1003, -8.6636) (-39.1671, -8.7182) (-39.2338, -8.7732) (-39.3002, -8.8285) (-39.3665, -8.8842) (-39.4326, -8.9404) (-39.4985, -8.9968) (-39.5642, -9.0537) (-39.6297, -9.1109) (-39.6951, -9.1685) (-39.7603, -9.2264) (-39.8253, -9.2847) (-39.8901, -9.3434) (-39.9547, -9.4024) (-40.0191, -9.4618) (-40.0706, -9.5095) (-40.109, -9.5455) (-40.1347, -9.5696) (-40.1475, -9.5816) knots 0 0 0 0 0 0 0.01428571 0.02857143 0.04285714 0.05714286 0.07142857 0.08571429 0.1 0.11428571 0.12857143 0.14285714 0.15714286 0.17142857 0.18571429 0.2 0.21428571 0.22857143 0.24285714 0.25714286 0.27142857 0.28571429 0.3 0.31428571 0.32857143 0.34285714 0.35714286 0.37142857 0.38571429 0.4 0.41428571 0.42857143 0.44285714 0.45714286 0.47142857 0.48571429 0.5 0.51428571 0.52857143 0.54285714 0.55714286 0.57142857 0.58571429 0.6 0.61428571 0.62857143 0.64285714 0.65714286 0.67142857 0.68571429 0.7 0.71428571 0.72857143 0.74285714 0.75714286 0.77142857 0.78571429 0.8 0.81428571 0.82857143 0.84285714 0.85714286 0.87142857 0.88571429 0.9 0.91428571 0.92857143 0.94285714 0.95714286 0.97142857 0.98571429 1 1 1 1 1 1
  arc A6 (-40.1475, -9.5816) -> (-39.5595, -11.7758) centre (0, 0) ccw
  spline S3 degree 5 poles (-39.5595, -11.7758) (-39.5424, -11.7798) (-39.5082, -11.7879) (-39.4569, -11.7998) (-39.3885, -11.8154) (-39.303, -11.8346) (-39.2175, -11.8534) (-39.132, -11.8718) (-39.0466, -11.8898) (-38.9612, -11.9074) (-38.8758, -11.9246) (-38.7904, -11.9414) (-38.7051, -11.9577) (-38.6198, -11.9737) (-38.5345, -11.9892) (-38.4492, -12.0044) (-38.364, -12.0191) (-38.2788, -12.0334) (-38.1937, -12.0473) (-38.1086, -12.0607) (-38.0235, -12.0737) (-37.9384, -12.0863) (-37.8535, -12.0985) (-37.7685, -12.1102) (-37.6836, -12.1215) (-37.5988, -12.1323) (-37.514, -12.1427) (-37.4292, -12.1526) (-37.3445, -12.1621) (-37.2599, -12.1711) (-37.1753, -12.1797) (-37.0908, -12.1878) (-37.0064, -12.1954) (-36.922, -12.2026) (-36.8377, -12.2092) (-36.7535, -12.2154) (-36.6693, -12.2211) (-36.5852, -12.2263) (-36.5012, -12.231) (-36.4173, -12.2353) (-36.3334, -12.239) (-36.2497, -12.2421) (-36.166, -12.2448) (-36.0824, -12.2469) (-35.999, -12.2484) (-35.9156, -12.2495) (-35.8323, -12.2499) (-35.7492, -12.2499) (-35.6661, -12.2493) (-35.5832, -12.2481) (-35.5004, -12.2463) (-35.4177, -12.2439) (-35.3352, -12.2408) (-35.2528, -12.2371) (-35.1705, -12.2327) (-35.0884, -12.2276) (-35.0065, -12.222) (-34.9246, -12.2159) (-34.8429, -12.2091) (-34.7614, -12.2015) (-34.6801, -12.1932) (-34.5991, -12.1838) (-34.5183, -12.1734) (-34.4378, -12.162) (-34.3576, -12.1496) (-34.2775, -12.1365) (-34.1976, -12.1229) (-34.1179, -12.1089) (-34.0383, -12.0941) (-33.9592, -12.0779) (-33.8808, -12.0596) (-33.8187, -12.0425) (-33.7726, -12.0281) (-33.7422, -12.0177) (-33.727, -12.0123) knots -1 -1 -1 -1 -1 -1 -0.98571429 -0.97142857 -0.95714286 -0.94285714 -0.92857143 -0.91428571 -0.9 -0.88571429 -0.87142857 -0.85714286 -0.84285714 -0.82857143 -0.81428571 -0.8 -0.78571429 -0.77142857 -0.75714286 -0.74285714 -0.72857143 -0.71428571 -0.7 -0.68571429 -0.67142857 -0.65714286 -0.64285714 -0.62857143 -0.61428571 -0.6 -0.58571429 -0.57142857 -0.55714286 -0.54285714 -0.52857143 -0.51428571 -0.5 -0.48571429 -0.47142857 -0.45714286 -0.44285714 -0.42857143 -0.41428571 -0.4 -0.38571429 -0.37142857 -0.35714286 -0.34285714 -0.32857143 -0.31428571 -0.3 -0.28571429 -0.27142857 -0.25714286 -0.24285714 -0.22857143 -0.21428571 -0.2 -0.18571429 -0.17142857 -0.15714286 -0.14285714 -0.12857143 -0.11428571 -0.1 -0.08571429 -0.07142857 -0.05714286 -0.04285714 -0.02857143 -0.01428571 0 0 0 0 0 0
  line L3 (-33.727, -12.0123) -> (-33.7161, -12.0084)
  arc A7 (-31.7138, -12.9058) -> (-33.7161, -12.0084) centre (-33.1842, -13.5041) ccw
  arc A8 (-31.7138, -12.9058) -> (-31.5508, -13.2993) centre (0, 0) ccw
  arc A9 (-32.3321, -15.3497) -> (-31.5508, -13.2993) centre (-33.0136, -13.9159) ccw
  line L4 (-32.3321, -15.3497) -> (-32.3425, -15.3546)
  spline S4 degree 5 poles (-32.3425, -15.3546) (-32.3571, -15.3615) (-32.386, -15.3757) (-32.4288, -15.3981) (-32.4847, -15.4299) (-32.5532, -15.4724) (-32.6205, -15.5169) (-32.6872, -15.5627) (-32.7536, -15.6091) (-32.8197, -15.656) (-32.8855, -15.7034) (-32.951, -15.7514) (-33.016, -15.8002) (-33.0805, -15.85) (-33.1444, -15.9007) (-33.2078, -15.9522) (-33.2708, -16.0046) (-33.3333, -16.0575) (-33.3956, -16.111) (-33.4575, -16.165) (-33.5191, -16.2195) (-33.5804, -16.2746) (-33.6413, -16.3302) (-33.7018, -16.3863) (-33.762, -16.4431) (-33.8218, -16.5004) (-33.8813, -16.5582) (-33.9405, -16.6165) (-33.9993, -16.6753) (-34.0578, -16.7345) (-34.1161, -16.7942) (-34.174, -16.8543) (-34.2316, -16.9149) (-34.2889, -16.9759) (-34.3459, -17.0374) (-34.4025, -17.0993) (-34.4589, -17.1616) (-34.515, -17.2243) (-34.5707, -17.2875) (-34.6262, -17.351) (-34.6814, -17.4149) (-34.7363, -17.4793) (-34.7909, -17.544) (-34.8453, -17.6091) (-34.8993, -17.6746) (-34.953, -17.7404) (-35.0065, -17.8067) (-35.0597, -17.8733) (-35.1126, -17.9402) (-35.1652, -18.0075) (-35.2175, -18.0752) (-35.2696, -18.1432) (-35.3214, -18.2115) (-35.3729, -18.2802) (-35.4241, -18.3492) (-35.475, -18.4186) (-35.5257, -18.4883) (-35.5761, -18.5583) (-35.6262, -18.6287) (-35.6761, -18.6993) (-35.7257, -18.7703) (-35.775, -18.8416) (-35.824, -18.9132) (-35.8728, -18.9852) (-35.9213, -19.0574) (-35.9695, -19.1299) (-36.0175, -19.2028) (-36.0652, -19.2759) (-36.1126, -19.3493) (-36.1598, -19.4231) (-36.2066, -19.4971) (-36.2439, -19.5565) (-36.2718, -19.6012) (-36.2903, -19.6311) (-36.2996, -19.6461) knots 0 0 0 0 0 0 0.01428571 0.02857143 0.04285714 0.05714286 0.07142857 0.08571429 0.1 0.11428571 0.12857143 0.14285714 0.15714286 0.17142857 0.18571429 0.2 0.21428571 0.22857143 0.24285714 0.25714286 0.27142857 0.28571429 0.3 0.31428571 0.32857143 0.34285714 0.35714286 0.37142857 0.38571429 0.4 0.41428571 0.42857143 0.44285714 0.45714286 0.47142857 0.48571429 0.5 0.51428571 0.52857143 0.54285714 0.55714286 0.57142857 0.58571429 0.6 0.61428571 0.62857143 0.64285714 0.65714286 0.67142857 0.68571429 0.7 0.71428571 0.72857143 0.74285714 0.75714286 0.77142857 0.78571429 0.8 0.81428571 0.82857143 0.84285714 0.85714286 0.87142857 0.88571429 0.9 0.91428571 0.92857143 0.94285714 0.95714286 0.97142857 0.98571429 1 1 1 1 1 1
  arc A10 (-36.2996, -19.6461) -> (-35.1638, -21.6133) centre (0, 0) ccw
  spline S5 degree 5 poles (-35.1638, -21.6133) (-35.1462, -21.6128) (-35.1111, -21.6117) (-35.0584, -21.6099) (-34.9883, -21.6073) (-34.9007, -21.6037) (-34.8133, -21.5998) (-34.726, -21.5954) (-34.6388, -21.5907) (-34.5518, -21.5856) (-34.4648, -21.5801) (-34.378, -21.5742) (-34.2914, -21.5679) (-34.2048, -21.5612) (-34.1184, -21.5542) (-34.0321, -21.5467) (-33.946, -21.5389) (-33.86, -21.5307) (-33.7742, -21.522) (-33.6885, -21.513) (-33.6029, -21.5035) (-33.5176, -21.4937) (-33.4323, -21.4834) (-33.3472, -21.4728) (-33.2623, -21.4617) (-33.1776, -21.4502) (-33.093, -21.4383) (-33.0085, -21.4259) (-32.9243, -21.4132) (-32.8402, -21.4) (-32.7563, -21.3864) (-32.6726, -21.3723) (-32.589, -21.3578) (-32.5057, -21.3429) (-32.4225, -21.3275) (-32.3395, -21.3117) (-32.2568, -21.2954) (-32.1742, -21.2787) (-32.0918, -21.2615) (-32.0097, -21.2438) (-31.9277, -21.2257) (-31.846, -21.2071) (-31.7645, -21.188) (-31.6832, -21.1684) (-31.6022, -21.1483) (-31.5214, -21.1277) (-31.4409, -21.1066) (-31.3605, -21.0851) (-31.2805, -21.063) (-31.2007, -21.0404) (-31.1211, -21.0172) (-31.0419, -20.9935) (-30.963, -20.9691) (-30.8844, -20.9442) (-30.8061, -20.9186) (-30.7281, -20.8925) (-30.6503, -20.8659) (-30.5729, -20.8388) (-30.4957, -20.8111) (-30.419, -20.7827) (-30.3426, -20.7536) (-30.2667, -20.7236) (-30.1914, -20.6926) (-30.1166, -20.6607) (-30.0423, -20.628) (-29.9684, -20.5947) (-29.8947, -20.5609) (-29.8213, -20.5266) (-29.7483, -20.4917) (-29.6761, -20.4557) (-29.605, -20.4177) (-29.5495, -20.3851) (-29.5088, -20.3592) (-29.482, -20.3413) (-29.4688, -20.3321) knots -1 -1 -1 -1 -1 -1 -0.98571429 -0.97142857 -0.95714286 -0.94285714 -0.92857143 -0.91428571 -0.9 -0.88571429 -0.87142857 -0.85714286 -0.84285714 -0.82857143 -0.81428571 -0.8 -0.78571429 -0.77142857 -0.75714286 -0.74285714 -0.72857143 -0.71428571 -0.7 -0.68571429 -0.67142857 -0.65714286 -0.64285714 -0.62857143 -0.61428571 -0.6 -0.58571429 -0.57142857 -0.55714286 -0.54285714 -0.52857143 -0.51428571 -0.5 -0.48571429 -0.47142857 -0.45714286 -0.44285714 -0.42857143 -0.41428571 -0.4 -0.38571429 -0.37142857 -0.35714286 -0.34285714 -0.32857143 -0.31428571 -0.3 -0.28571429 -0.27142857 -0.25714286 -0.24285714 -0.22857143 -0.21428571 -0.2 -0.18571429 -0.17142857 -0.15714286 -0.14285714 -0.12857143 -0.11428571 -0.1 -0.08571429 -0.07142857 -0.05714286 -0.04285714 -0.02857143 -0.01428571 0 0 0 0 0 0
  line L5 (-29.4688, -20.3321) -> (-29.4592, -20.3256)
  arc A11 (-27.2929, -20.6741) -> (-29.4592, -20.3256) centre (-28.5583, -21.6327) ccw
  arc A12 (-27.2929, -20.6741) -> (-27.0336, -21.0121) centre (0, 0) ccw
  arc A13 (-27.2576, -23.1948) -> (-27.0336, -21.0121) centre (-28.287, -21.9863) ccw
  line L6 (-27.2576, -23.1948) -> (-27.2664, -23.2023)
  spline S6 degree 5 poles (-27.2664, -23.2023) (-27.2787, -23.2127) (-27.3029, -23.2339) (-27.3385, -23.2666) (-27.3843, -23.3118) (-27.4394, -23.3706) (-27.4929, -23.431) (-27.5455, -23.4925) (-27.5976, -23.5545) (-27.6493, -23.6169) (-27.7006, -23.6797) (-27.7515, -23.743) (-27.8016, -23.807) (-27.851, -23.8718) (-27.8997, -23.9373) (-27.9475, -24.0035) (-27.9948, -24.0703) (-28.0415, -24.1377) (-28.0878, -24.2055) (-28.1337, -24.2736) (-28.1791, -24.3422) (-28.224, -24.4113) (-28.2684, -24.4807) (-28.3124, -24.5507) (-28.3558, -24.6211) (-28.3988, -24.6919) (-28.4413, -24.7631) (-28.4833, -24.8347) (-28.5249, -24.9067) (-28.5661, -24.9791) (-28.6069, -25.0518) (-28.6473, -25.1249) (-28.6873, -25.1983) (-28.7268, -25.2721) (-28.766, -25.3462) (-28.8047, -25.4206) (-28.843, -25.4954) (-28.8809, -25.5705) (-28.9185, -25.646) (-28.9556, -25.7217) (-28.9924, -25.7978) (-29.0287, -25.8741) (-29.0647, -25.9508) (-29.1004, -26.0277) (-29.1356, -26.1049) (-29.1705, -26.1825) (-29.205, -26.2603) (-29.2391, -26.3383) (-29.2729, -26.4167) (-29.3063, -26.4953) (-29.3393, -26.5742) (-29.372, -26.6534) (-29.4043, -26.7328) (-29.4363, -26.8125) (-29.4679, -26.8924) (-29.4992, -26.9726) (-29.5301, -27.053) (-29.5606, -27.1337) (-29.5909, -27.2147) (-29.6207, -27.2958) (-29.6502, -27.3772) (-29.6794, -27.4589) (-29.7082, -27.5407) (-29.7367, -27.6228) (-29.7649, -27.7051) (-29.7927, -27.7877) (-29.8202, -27.8705) (-29.8473, -27.9534) (-29.8741, -28.0366) (-29.9006, -28.1201) (-29.9267, -28.2037) (-29.9474, -28.2708) (-29.9627, -28.3212) (-29.9728, -28.3548) (-29.9779, -28.3717) knots 0 0 0 0 0 0 0.01428571 0.02857143 0.04285714 0.05714286 0.07142857 0.08571429 0.1 0.11428571 0.12857143 0.14285714 0.15714286 0.17142857 0.18571429 0.2 0.21428571 0.22857143 0.24285714 0.25714286 0.27142857 0.28571429 0.3 0.31428571 0.32857143 0.34285714 0.35714286 0.37142857 0.38571429 0.4 0.41428571 0.42857143 0.44285714 0.45714286 0.47142857 0.48571429 0.5 0.51428571 0.52857143 0.54285714 0.55714286 0.57142857 0.58571429 0.6 0.61428571 0.62857143 0.64285714 0.65714286 0.67142857 0.68571429 0.7 0.71428571 0.72857143 0.74285714 0.75714286 0.77142857 0.78571429 0.8 0.81428571 0.82857143 0.84285714 0.85714286 0.87142857 0.88571429 0.9 0.91428571 0.92857143 0.94285714 0.95714286 0.97142857 0.98571429 1 1 1 1 1 1
  arc A14 (-29.9779, -28.3717) -> (-28.3717, -29.9779) centre (0, 0) ccw